Autodesk Fusion 360 part; units mm, degrees
note: some values were not read from the file. Chosen so that the rebuilt part matches the saved one: that a step has no effect; which bodies a step acts on.
(part 2 of 3)
  spline S56 degree 5 poles (56.3388, 91.0993) (56.4452, 91.2557) (56.6813, 91.5544) (57.0997, 91.9524) (57.7606, 92.3569) (58.6747, 92.6057) (59.5849, 92.5729) (60.4007, 92.2578) (61.0421, 91.6864) (61.4504, 90.9158) (61.5889, 90.0247) (61.4439, 89.103) (61.0258, 88.2423) (60.3712, 87.5263) (59.5452, 87.0208) (58.6311, 86.772) (57.7208, 86.8047) (56.905, 87.1199) (56.2637, 87.6913) (55.8554, 88.4618) (55.7168, 89.353) (55.8328, 90.0903) (56.0427, 90.6159) (56.2324, 90.9429) (56.3388, 91.0993) knots 0 0 0 0 0 0 0.05 0.1 0.15 0.2 0.25 0.3 0.35 0.4 0.45 0.5 0.55 0.6 0.65 0.7 0.75 0.8 0.85 0.9 0.95 1 1 1 1 1 1
  spline S57 degree 5 poles (56.8751, 97.0852) (56.9558, 96.9232) (57.0765, 96.5874) (57.1351, 96.0509) (56.9827, 95.2754) (56.5, 94.2116) (55.843, 93.064) (55.1256, 91.8622) (54.4274, 90.6693) (53.766, 89.5941) (53.1219, 88.7638) (52.4603, 88.2976) (51.7518, 88.283) (50.9983, 88.7439) (50.2411, 89.6329) (49.5446, 90.8558) (48.9852, 92.2891) (48.6393, 93.7983) (48.5705, 95.257) (48.8189, 96.5627) (49.3981, 97.6352) (50.2913, 98.4191) (51.4468, 98.8843) (52.7731, 99.028) (54.135, 98.8762) (55.3803, 98.4726) (56.1682, 97.9896) (56.5924, 97.5594) (56.7944, 97.2472) (56.8751, 97.0852) knots 0 0 0 0 0 0 0.04 0.08 0.12 0.16 0.2 0.24 0.28 0.32 0.36 0.4 0.44 0.48 0.52 0.56 0.6 0.64 0.68 0.72 0.76 0.8 0.84 0.88 0.92 0.96 1 1 1 1 1 1
  spline S58 degree 5 poles (71.8814, 95.613) (71.9027, 95.4116) (71.8949, 95.0024) (71.7344, 94.3767) (71.2451, 93.5503) (70.2783, 92.62) (69.0821, 91.8793) (67.7798, 91.4005) (66.4658, 91.2268) (65.1864, 91.362) (63.9606, 91.7809) (62.7952, 92.4363) (61.7022, 93.2674) (60.7152, 94.2071) (59.9065, 95.1895) (59.3667, 96.1526) (59.1837, 97.0411) (59.424, 97.8085) (60.1077, 98.4213) (61.2044, 98.8582) (62.6448, 99.107) (64.3273, 99.1623) (66.1266, 99.0235) (67.9002, 98.6914) (69.4995, 98.1694) (70.7863, 97.4683) (71.4751, 96.7812) (71.7673, 96.2113) (71.8601, 95.8145) (71.8814, 95.613) knots 0 0 0 0 0 0 0.04 0.08 0.12 0.16 0.2 0.24 0.28 0.32 0.36 0.4 0.44 0.48 0.52 0.56 0.6 0.64 0.68 0.72 0.76 0.8 0.84 0.88 0.92 0.96 1 1 1 1 1 1
  spline S59 degree 5 poles (93.1796, 92.4377) (92.9012, 92.2188) (92.3428, 91.7857) (91.5103, 91.1539) (90.4378, 90.3537) (89.1797, 89.4222) (87.9931, 88.5509) (86.8537, 87.7371) (85.7383, 86.994) (84.6458, 86.3666) (83.5926, 85.9228) (82.5959, 85.7326) (81.6625, 85.8525) (80.7707, 86.3039) (79.8819, 87.0726) (78.9677, 88.1162) (78.0294, 89.3696) (77.1277, 90.7501) (76.3717, 92.1664) (75.8904, 93.5293) (75.8092, 94.7623) (76.2256, 95.8109) (77.1816, 96.656) (78.6644, 97.3069) (80.6168, 97.79) (82.9427, 98.1396) (85.515, 98.3871) (88.1823, 98.5517) (90.7746, 98.6284) (93.1172, 98.5921) (95.0483, 98.409) (96.4351, 98.0455) (97.1913, 97.4789) (97.2921, 96.7056) (96.798, 95.7541) (95.8395, 94.6799) (94.8313, 93.7751) (94.0132, 93.0995) (93.458, 92.6567) (93.1796, 92.4377) knots 0 0 0 0 0 0 0.028571 0.057143 0.085714 0.114286 0.142857 0.171429 0.2 0.228571 0.257143 0.285714 0.314286 0.342857 0.371429 0.4 0.428571 0.457143 0.485714 0.514286 0.542857 0.571429 0.6 0.628571 0.657143 0.685714 0.714286 0.742857 0.771429 0.8 0.828571 0.857143 0.885714 0.914286 0.942857 0.971429 1 1 1 1 1 1
  line L0 (0, 0) -> (100, 0)
  line L1 (100, 0) -> (100, 100)
  line L2 (100, 100) -> (0, 100)
  line L3 (0, 100) -> (0, 0)
  point P0 (79.6579, 4.5542)
  point P1 (83.6873, 0.8119)
  point P2 (76.3709, 0.506)
  point P3 (52.7695, 4.9862)
  point P4 (57.3318, 2.811)
  point P5 (50.8771, 0.554)
  point P6 (96.4606, 14.0148)
  point P7 (98.7941, 14.2851)
  point P8 (98.8112, 7.9358)
  point P9 (92.875, 1.5897)
  point P10 (86.8955, 1.8956)
  point P11 (46.6878, 15.1123)
  point P12 (48.5368, 10.226)
  point P13 (44.8148, 3.7468)
  point P14 (39.7202, 1.5716)
  point P15 (53.9319, 10.5579)
  point P16 (52.8052, 6.5669)
  point P17 (50.0726, 10.7891)
  point P18 (80.2047, 15.9155)
  point P19 (87.817, 16.1625)
  point P20 (88.2258, 8.7488)
  point P21 (80.5937, 6.4154)
  point P22 (67.9071, 12.0123)
  point P23 (72.899, 13.9305)
  point P24 (73.8805, 11.2313)
  point P25 (70.5305, 5.4026)
  point P26 (65.0899, 1.6603)
  point P27 (60.2064, 12.5056)
  point P28 (61.4147, 5.5204)
  point P29 (60.8831, 1.6099)
  point P30 (58.7258, 3.8669)
  point P31 (55.2901, 10.0331)
  point P32 (64.2148, 19.7302)
  point P33 (68.5192, 18.2733)
  point P34 (71.0087, 16.4698)
  point P35 (67.2346, 13.716)
  point P36 (61.5672, 14.2597)
  point P37 (39.3527, 17.9605)
  point P38 (43.7129, 16.5883)
  point P39 (40.5628, 9.3364)
  point P40 (33.3674, 2.2747)
  point P41 (31.3901, 20.6466)
  point P42 (30.1837, 10.7278)
  point P43 (23.6179, 2.2941)
  point P44 (24.7173, 24.277)
  point P45 (28.0018, 24.0715)
  point P46 (23.6955, 13.0275)
  point P47 (15.6156, 3.1087)
  point P48 (19.1559, 23.32)
  point P49 (15.0058, 12.9492)
  point P50 (6.1601, 2.8249)
  point P51 (2.1097, 10.5786)
  point P52 (50.3349, 28.7902)
  point P53 (54.7428, 27.0564)
  point P54 (58.5479, 22.4518)
  point P55 (58.378, 19.3657)
  point P56 (54.9409, 17.4108)
  point P57 (51.2592, 16.9047)
  point P58 (48.2836, 17.8001)
  point P59 (46.6034, 18.5729)
  point P60 (77.4266, 28.2267)
  point P61 (80.5194, 27.0023)
  point P62 (82.2807, 22.8761)
  point P63 (79.1441, 17.9256)
  point P64 (74.5854, 16.6476)
  point P65 (73.3675, 17.4831)
  point P66 (71.9781, 29.9866)
  point P67 (73.0873, 23.6564)
  point P68 (69.5529, 19.8978)
  point P69 (15.057, 28.1496)
  point P70 (9.8735, 23.0445)
  point P71 (1.673, 21.0503)
  point P72 (91.0208, 30.4127)
  point P73 (95.3534, 23.8248)
  point P74 (95.7627, 17.1433)
  point P75 (89.3915, 18.5135)
  point P76 (84.9158, 23.217)
  point P77 (33.9696, 30.4461)
  point P78 (41.5842, 31.0743)
  point P79 (44.4066, 24.3171)
  point P80 (39.0181, 20.9457)
  point P81 (33.1247, 23.6126)
  point P82 (30.8652, 26.2228)
  point P83 (67.2233, 32.9776)
  point P84 (68.1538, 32.1594)
  point P85 (67.3369, 26.8095)
  point P86 (64.1417, 21.9362)
  point P87 (61.1337, 23.7625)
  point P88 (57.8109, 34.4437)
  point P89 (63.6671, 35.1504)
  point P90 (62.0694, 30.3434)
  point P91 (55.9996, 29.2565)
  point P92 (98.029, 32.816)
  point P93 (99.5699, 25.3331)
  point P94 (99.5529, 17.9925)
  point P95 (96.81, 24.4037)
  point P96 (16.4842, 40.0903)
  point P97 (17.8044, 42.8105)
  point P98 (19.0706, 42.1969)
  point P99 (23.606, 35.4655)
  point P100 (27.0735, 29.1141)
  point P101 (24.3862, 28.0614)
  point P102 (21.0871, 27.3883)
  point P103 (17.4249, 30.1227)
  point P104 (12.2185, 34.2787)
  point P105 (6.5411, 27.4672)
  point P106 (1.3576, 28.0394)
  point P107 (83.2708, 40.527)
  point P108 (86.6058, 36.7601)
  point P109 (85.565, 30.6337)
  point P110 (81.7651, 29.5421)
  point P111 (77.9962, 41.0906)
  point P112 (79.1698, 35.5905)
  point P113 (76.9524, 30.8901)
  point P114 (72.829, 32.0389)
  point P115 (70.1115, 33.6302)
  point P116 (7.7831, 51.8118)
  point P117 (14.5473, 46.1719)
  point P118 (13.9992, 42.5886)
  point P119 (7.2333, 38.0106)
  point P120 (1.5559, 46.472)
  point P121 (93.088, 42.9022)
  point P122 (94.9293, 37.8383)
  point P123 (94.0768, 34.227)
  point P124 (91.268, 33.3354)
  point P125 (88.2424, 37.4838)
  point P126 (36.6083, 39.904)
  point P127 (32.9758, 32.7946)
  point P128 (25.8067, 36.1809)
  point P129 (45.0765, 42.7464)
  point P130 (50.2538, 36.7891)
  point P131 (50.7512, 33.3436)
  point P132 (48.9583, 32.0429)
  point P133 (43.4327, 33.3262)
  point P134 (39.4507, 39.8074)
  point P135 (99.5711, 37.3522)
  point P136 (98.0302, 35.0244)
  point P137 (96.14, 37.703)
  point P138 (59.3387, 46.6587)
  point P139 (60.8929, 46.1985)
  point P140 (61.3985, 42.1766)
  point P141 (57.6584, 36.4209)
  point P142 (52.7347, 37.7138)
  point P143 (74.3353, 44.1904)
  point P144 (71.7761, 39.0436)
  point P145 (67.896, 35.5105)
  point P146 (65.6687, 36.7939)
  point P147 (63.5526, 41.8429)
  point P148 (96.04, 49.1785)
  point P149 (99.1607, 45.7878)
  point P150 (97.2704, 41.6705)
  point P151 (93.8882, 44.4065)
  point P152 (44.4535, 58.6502)
  point P153 (50.6119, 53.9651)
  point P154 (52.7715, 45.7846)
  point P155 (45.4083, 45.526)
  point P156 (79.0137, 56.0424)
  point P157 (82.0596, 58.6914)
  point P158 (86.8617, 53.6865)
  point P159 (89.9799, 48.3562)
  point P160 (87.3322, 45.7144)
  point P161 (83.0298, 43.5257)
  point P162 (79.475, 43.9658)
  point P163 (77.0992, 46.0034)
  point P164 (40.3762, 58.1751)
  point P165 (39.3724, 53.1339)
  point P166 (37.5699, 47.4134)
  point P167 (29.8388, 45.7456)
  point P168 (21.6709, 45.3675)
  point P169 (69.9242, 53.2274)
  point P170 (73.9562, 50.2914)
  point P171 (68.183, 47.579)
  point P172 (62.891, 47.7375)
  point P173 (25.9752, 54.1385)
  point P174 (36.1891, 59.6447)
  point P175 (28.5971, 52.2783)
  point P176 (18.5959, 46.1828)
  point P177 (17.8238, 47.0459)
  point P178 (51.7742, 62.944)
  point P179 (58.7457, 63.9787)
  point P180 (62.7216, 59.0715)
  point P181 (61.8264, 52.1149)
  point P182 (59.0452, 49.7589)
  point P183 (52.4674, 55.2104)
  point P184 (76.4459, 63.7521)
  point P185 (76.9263, 58.2048)
  point P186 (70.7568, 55.3301)
  point P187 (65.8459, 59.6129)
  point P188 (30.2252, 66.8582)
  point P189 (32.7416, 64.9211)
  point P190 (26.95, 56.7534)
  point P191 (25.1065, 65.5592)
  point P192 (22.1685, 57.8836)
  point P193 (16.3207, 49.4431)
  point P194 (9.6797, 53.9745)
  point P195 (97.2127, 66.1551)
  point P196 (98.872, 59.495)
  point P197 (95.7513, 51.889)
  point P198 (89.2508, 55.6261)
  point P199 (78.7543, 79.2824)
  point P200 (81.557, 81.7992)
  point P201 (88.0419, 75.3523)
  point P202 (88.237, 65.7773)
  point P203 (81.9734, 63.1837)
  point P204 (78.4471, 66.0821)
  point P205 (16.0982, 74.0254)
  point P206 (11.0462, 63.9161)
  point P207 (1.4654, 60.7724)
  point P208 (1.4636, 64.0146)
  point P209 (60.0445, 76.0097)
  point P210 (68.0434, 77.5129)
  point P211 (73.3977, 72.7761)
  point P212 (68.4387, 67.3518)
  point P213 (60.3971, 66.8153)
  point P214 (25.6397, 89.5124)
  point P215 (29.4587, 76.9092)
  point P216 (29.4909, 70.2325)
  point P217 (26.6373, 69.7404)
  point P218 (19.6178, 76.2868)
  point P219 (44.314, 71.0287)
  point P220 (44.5931, 62.6999)
  point P221 (42.9899, 61.8846)
  point P222 (41.6871, 61.6373)
  point P223 (39.3087, 62.9052)
  point P224 (34.9761, 66.0859)
  point P225 (32.4275, 74.6996)
  point P226 (52.3135, 78.1832)
  point P227 (54.4898, 71.1149)
  point P228 (50.5582, 66.1591)
  point P229 (46.4172, 72.2548)
  point P230 (94.8024, 80.3857)
  point P231 (98.768, 72.2616)
  point P232 (97.1087, 69.6161)
  point P233 (90.4132, 76.2607)
  point P234 (99.3391, 85.828)
  point P235 (95.3735, 82.3698)
  point P236 (52.493, 86.1688)
  point P237 (56.1856, 85.8873)
  point P238 (59.5862, 82.883)
  point P239 (58.146, 78.2422)
  point P240 (53.2824, 80.0373)
  point P241 (68.7729, 89.4265)
  point P242 (75.3354, 87.0977)
  point P243 (76.1801, 81.8417)
  point P244 (68.9433, 80.107)
  point P245 (62.3846, 83.2446)
  point P246 (15.8973, 91.7004)
  point P247 (7.2818, 78.7031)
  point P248 (2.228, 84.9448)
  point P249 (10.8389, 98.0538)
  point P250 (47.5058, 86.5545)
  point P251 (45.046, 84.5348)
  point P252 (37.3316, 84.77)
  point P253 (28.1564, 91.9777)
  point P254 (24.7262, 98.0892)
  point P255 (34.0446, 98.2008)
  point P256 (60.4137, 92.1585)
  point P257 (60.9669, 88.2783)
  point P258 (56.892, 87.2191)
  point P259 (55.1789, 91.9477)
  point P260 (52.0396, 88.3491)
  point P261 (48.755, 93.4866)
  point P262 (51.419, 98.7862)
  point P263 (67.9939, 91.5348)
  point P264 (61.7267, 93.2966)
  point P265 (59.3479, 97.3748)
  point P266 (65.1388, 99.0758)
  point P267 (86.4841, 87.5)
  point P268 (82.3055, 85.8154)
  point P269 (78.6581, 88.5545)
  point P270 (75.983, 94.9616)
  point P271 (86.3259, 98.4244)
  point P272 (97.1452, 97.1602)
move_body "Move1" bodies 2 to x (1, 0, 0) y (0, 1, 0) z (0, 0, 1) at (30, 0, 0)
extrude "Extrude12" cut sketch "Voronoi - Sketch2" along normal blind 100 contours S9 | S10 | S11 | S12 | S16 | S18 | S22 | S23 | S26 | S28 | S29 | S34 | S36 | S38 | S41 | S42 | S45 | S47 | S48 | S54 | S55 bodies 2
sketch "Voronoi - Sketch3" plane through (0, 0, 0) normal (0, 0, 1) x (1, 0, 0)
  spline S0 degree 5 poles (17.018, 3.2698) (17.8759, 3.2327) (19.5931, 3.1438) (22.1324, 2.9685) (25.2811, 2.6617) (28.4421, 2.1957) (30.5103, 1.6941) (31.2641, 1.2063) (30.6122, 0.7793) (28.634, 0.453) (25.5432, 0.2578) (21.6516, 0.2133) (17.3358, 0.3263) (13.0049, 0.5879) (9.0689, 0.9714) (5.908, 1.4374) (3.8397, 1.9391) (3.0859, 2.4269) (3.7378, 2.8538) (5.716, 3.1802) (8.8068, 3.3754) (11.9201, 3.4109) (14.446, 3.3667) (16.1602, 3.307) (17.018, 3.2698) knots 0 0 0 0 0 0 0.05 0.1 0.15 0.2 0.25 0.3 0.35 0.4 0.45 0.5 0.55 0.6 0.65 0.7 0.75 0.8 0.85 0.9 0.95 1 1 1 1 1 1
  spline S1 degree 5 poles (72.5597, 3.806) (72.5934, 4.0043) (72.6951, 4.4023) (72.9489, 4.9941) (73.475, 5.7348) (74.3766, 6.4919) (75.4317, 7.0052) (76.5375, 7.2209) (77.5882, 7.1125) (78.4845, 6.6913) (79.1407, 6.0037) (79.491, 5.1203) (79.4962, 4.128) (79.1514, 3.1214) (78.4938, 2.1955) (77.5922, 1.4385) (76.5371, 0.9251) (75.4313, 0.7094) (74.3806, 0.8179) (73.4843, 1.2391) (72.8281, 1.9267) (72.5478, 2.6334) (72.493, 3.2124) (72.526, 3.6076) (72.5597, 3.806) knots 0 0 0 0 0 0 0.05 0.1 0.15 0.2 0.25 0.3 0.35 0.4 0.45 0.5 0.55 0.6 0.65 0.7 0.75 0.8 0.85 0.9 0.95 1 1 1 1 1 1
  spline S2 degree 5 poles (84.9841, 9.4583) (85.2417, 9.591) (85.773, 9.817) (86.6121, 10.031) (87.7977, 10.0538) (89.3704, 9.67) (91.0179, 8.9401) (92.7087, 7.9558) (94.3794, 6.82) (95.9099, 5.6313) (97.1436, 4.4775) (97.9224, 3.4322) (98.1159, 2.5505) (97.6531, 1.8644) (96.5566, 1.3779) (94.9239, 1.0767) (92.9034, 0.9392) (90.6733, 0.9473) (88.4208, 1.0964) (86.3194, 1.4085) (84.5195, 1.919) (83.1417, 2.6602) (82.2682, 3.6431) (81.9355, 4.8435) (82.122, 6.1788) (82.7534, 7.5117) (83.534, 8.4519) (84.2276, 9.0208) (84.7265, 9.3256) (84.9841, 9.4583) knots 0 0 0 0 0 0 0.04 0.08 0.12 0.16 0.2 0.24 0.28 0.32 0.36 0.4 0.44 0.48 0.52 0.56 0.6 0.64 0.68 0.72 0.76 0.8 0.84 0.88 0.92 0.96 1 1 1 1 1 1
  spline S3 degree 5 poles (3.4341, 11.1117) (3.6227, 11.2638) (4.0513, 11.5485) (4.8404, 11.9144) (6.1468, 12.2844) (8.0932, 12.6168) (10.2402, 12.9058) (12.4865, 13.2242) (14.7565, 13.596) (17.0129, 13.9632) (19.24, 14.2194) (21.4267, 14.2405) (23.5492, 13.9177) (25.556, 13.1869) (27.347, 12.0663) (28.7682, 10.6723) (29.6519, 9.1712) (29.8501, 7.7412) (29.2677, 6.5339) (27.9038, 5.6283) (25.8396, 5.0394) (23.2145, 4.7403) (20.2064, 4.6793) (17.0113, 4.7989) (13.8229, 5.0528) (10.8118, 5.4269) (8.1221, 5.9283) (5.8717, 6.5707) (4.1503, 7.3615) (3.0188, 8.2864) (2.5076, 9.2982) (2.593, 10.0964) (2.9197, 10.6362) (3.2455, 10.9597) (3.4341, 11.1117) knots 0 0 0 0 0 0 0.033333 0.066667 0.1 0.133333 0.166667 0.2 0.233333 0.266667 0.3 0.333333 0.366667 0.4 0.433333 0.466667 0.5 0.533333 0.566667 0.6 0.633333 0.666667 0.7 0.733333 0.766667 0.8 0.833333 0.866667 0.9 0.933333 0.966667 1 1 1 1 1 1
  spline S4 degree 5 poles (58.3825, 7.7649) (58.3025, 8.0979) (58.1596, 8.7676) (57.9974, 9.7704) (57.8928, 11.051) (57.9754, 12.423) (58.2988, 13.4519) (58.8841, 14.0645) (59.7367, 14.2533) (60.8405, 14.0911) (62.1601, 13.6923) (63.6425, 13.1808) (65.2192, 12.6587) (66.8064, 12.1663) (68.311, 11.6809) (69.6388, 11.147) (70.7033, 10.4969) (71.4334, 9.6746) (71.7826, 8.661) (71.7356, 7.4894) (71.303, 6.2268) (70.5199, 4.961) (69.442, 3.7856) (68.1439, 2.7854) (66.7121, 2.0314) (65.2357, 1.5806) (63.7983, 1.473) (62.4696, 1.7305) (61.2961, 2.3541) (60.297, 3.3226) (59.4752, 4.5928) (58.955, 5.7982) (58.6395, 6.7693) (58.4625, 7.4319) (58.3825, 7.7649) knots 0 0 0 0 0 0 0.033333 0.066667 0.1 0.133333 0.166667 0.2 0.233333 0.266667 0.3 0.333333 0.366667 0.4 0.433333 0.466667 0.5 0.533333 0.566667 0.6 0.633333 0.666667 0.7 0.733333 0.766667 0.8 0.833333 0.866667 0.9 0.933333 0.966667 1 1 1 1 1 1
  spline S5 degree 5 poles (36.564, 13.7854) (36.7145, 13.9752) (37.0446, 14.3355) (37.6279, 14.8158) (38.5691, 15.3327) (39.9402, 15.7841) (41.4046, 16.0661) (42.8601, 16.2146) (44.2264, 16.2715) (45.4689, 16.2809) (46.5889, 16.2788) (47.6106, 16.2815) (48.5701, 16.2764) (49.5027, 16.2061) (50.4335, 15.9774) (51.3692, 15.4979) (52.2923, 14.7023) (53.1497, 13.5903) (53.8614, 12.2209) (54.3368, 10.6884) (54.4893, 9.1031) (54.2505, 7.5721) (53.5872, 6.1763) (52.5087, 4.9597) (51.0576, 3.9408) (49.3035, 3.1191) (47.3359, 2.4837) (45.2574, 2.0206) (43.1772, 1.7205) (41.204, 1.587) (39.4376, 1.6317) (37.9592, 1.8694) (36.8226, 2.3136) (36.0452, 2.9714) (35.5969, 3.8387) (35.3967, 4.8964) (35.3446, 6.1125) (35.3513, 7.4436) (35.3659, 8.8373) (35.4104, 10.2332) (35.5552, 11.5685) (35.822, 12.5416) (36.142, 13.1965) (36.4136, 13.5955) (36.564, 13.7854) knots 0 0 0 0 0 0 0.025 0.05 0.075 0.1 0.125 0.15 0.175 0.2 0.225 0.25 0.275 0.3 0.325 0.35 0.375 0.4 0.425 0.45 0.475 0.5 0.525 0.55 0.575 0.6 0.625 0.65 0.675 0.7 0.725 0.75 0.775 0.8 0.825 0.85 0.875 0.9 0.925 0.95 0.975 1 1 1 1 1 1
  spline S6 degree 5 poles (74.5422, 18.1253) (74.6384, 18.3623) (74.8439, 18.8297) (75.1897, 19.5085) (75.721, 20.3642) (76.4882, 21.3545) (77.3417, 22.2742) (78.2583, 23.1294) (79.2059, 23.9145) (80.14, 24.6034) (81.0007, 25.1405) (81.7292, 25.4593) (82.286, 25.5031) (82.6664, 25.2427) (82.9237, 24.7009) (83.1438, 23.9374) (83.411, 23.0254) (83.7715, 22.0283) (84.21, 20.9833) (84.6733, 19.9107) (85.0856, 18.8196) (85.3681, 17.7149) (85.4548, 16.6032) (85.314, 15.5007) (84.9458, 14.4318) (84.3721, 13.4247) (83.6288, 12.508) (82.7584, 11.7072) (81.8004, 11.0405) (80.7869, 10.5171) (79.7459, 10.1415) (78.7033, 9.9162) (77.6852, 9.8452) (76.7201, 9.9367) (75.841, 10.2066) (75.0814, 10.6713) (74.4717, 11.3399) (74.0349, 12.2084) (73.7824, 13.2506) (73.7141, 14.4205) (73.8221, 15.6628) (74.0385, 16.6689) (74.2668, 17.4076) (74.4461, 17.8883) (74.5422, 18.1253) knots 0 0 0 0 0 0 0.025 0.05 0.075 0.1 0.125 0.15 0.175 0.2 0.225 0.25 0.275 0.3 0.325 0.35 0.375 0.4 0.425 0.45 0.475 0.5 0.525 0.55 0.575 0.6 0.625 0.65 0.675 0.7 0.725 0.75 0.775 0.8 0.825 0.85 0.875 0.9 0.925 0.95 0.975 1 1 1 1 1 1
  spline S7 degree 5 poles (60.7414, 19.3241) (60.802, 19.5667) (60.9786, 20.0469) (61.4066, 20.7403) (62.2786, 21.5665) (63.7567, 22.338) (65.4744, 22.772) (67.2645, 22.8211) (68.9554, 22.4733) (70.3875, 21.7638) (71.4241, 20.7679) (71.9612, 19.5873) (71.9383, 18.3386) (71.3503, 17.142) (70.2604, 16.1092) (68.7823, 15.3377) (67.0646, 14.9037) (65.2745, 14.8546) (63.5836, 15.2023) (62.1515, 15.9119) (61.1149, 16.9078) (60.6853, 17.8523) (60.615, 18.5913) (60.6808, 19.0815) (60.7414, 19.3241) knots 0 0 0 0 0 0 0.05 0.1 0.15 0.2 0.25 0.3 0.35 0.4 0.45 0.5 0.55 0.6 0.65 0.7 0.75 0.8 0.85 0.9 0.95 1 1 1 1 1 1
  spline S8 degree 5 poles (92.8632, 20.9454) (93.1944, 20.8939) (93.8613, 20.7346) (94.8595, 20.3297) (96.122, 19.4813) (97.4362, 18.0178) (98.3567, 16.2984) (98.7876, 14.4901) (98.6777, 12.7661) (98.0381, 11.2894) (96.9402, 10.2014) (95.497, 9.6112) (93.8507, 9.5844) (92.1587, 10.1308) (90.5805, 11.1913) (89.2664, 12.6547) (88.3458, 14.3742) (87.9149, 16.1824) (88.0248, 17.9065) (88.6644, 19.3831) (89.7624, 20.4711) (90.9169, 20.9433) (91.8742, 21.0439) (92.532, 20.997) (92.8632, 20.9454) knots 0 0 0 0 0 0 0.05 0.1 0.15 0.2 0.25 0.3 0.35 0.4 0.45 0.5 0.55 0.6 0.65 0.7 0.75 0.8 0.85 0.9 0.95 1 1 1 1 1 1
  spline S9 degree 5 poles (10.9889, 20.653) (11.1252, 21.0131) (11.4462, 21.7388) (12.0668, 22.8271) (13.1345, 24.2083) (14.7348, 25.6557) (16.4417, 26.6835) (18.0876, 27.1857) (19.5121, 27.1031) (20.5787, 26.4389) (21.1878, 25.267) (21.2798, 23.71) (20.8405, 21.9239) (19.9064, 20.0809) (18.5717, 18.3544) (16.9714, 16.907) (15.2646, 15.8792) (13.6187, 15.377) (12.1941, 15.4596) (11.1276, 16.1238) (10.5185, 17.2957) (10.4448, 18.5412) (10.6287, 19.5786) (10.8527, 20.293) (10.9889, 20.653) knots 0 0 0 0 0 0 0.05 0.1 0.15 0.2 0.25 0.3 0.35 0.4 0.45 0.5 0.55 0.6 0.65 0.7 0.75 0.8 0.85 0.9 0.95 1 1 1 1 1 1
  spline S10 degree 5 poles (85.1604, 28.0531) (85.2638, 28.1855) (85.5042, 28.4325) (85.9654, 28.7455) (86.7772, 29.0378) (88.089, 29.1968) (89.6454, 29.1705) (91.3697, 28.9889) (93.1593, 28.6831) (94.8801, 28.275) (96.38, 27.7774) (97.5114, 27.2005) (98.1525, 26.5559) (98.2265, 25.8617) (97.7284, 25.1481) (96.7308, 24.4586) (95.3538, 23.8433) (93.744, 23.3533) (92.0505, 23.0347) (90.4014, 22.9231) (88.8837, 23.0378) (87.5551, 23.3818) (86.452, 23.9403) (85.5977, 24.6796) (85.0103, 25.5461) (84.7124, 26.4629) (84.725, 27.1657) (84.8838, 27.6382) (85.057, 27.9207) (85.1604, 28.0531) knots 0 0 0 0 0 0 0.04 0.08 0.12 0.16 0.2 0.24 0.28 0.32 0.36 0.4 0.44 0.48 0.52 0.56 0.6 0.64 0.68 0.72 0.76 0.8 0.84 0.88 0.92 0.96 1 1 1 1 1 1
  spline S11 degree 5 poles (38.1151, 22.7911) (38.0638, 23.1142) (38.0024, 23.7754) (38.0359, 24.7965) (38.3318, 26.1516) (39.0774, 27.671) (40.1234, 28.8647) (41.3699, 29.6101) (42.7004, 29.8269) (43.9882, 29.4975) (45.1075, 28.6628) (45.9453, 27.4088) (46.4136, 25.8564) (46.4623, 24.1519) (46.0925, 22.458) (45.3469, 20.9386) (44.3009, 19.7449) (43.0543, 18.9995) (41.7239, 18.7827) (40.4361, 19.1121) (39.3168, 19.9468) (38.6465, 20.95) (38.3101, 21.8367) (38.1664, 22.468) (38.1151, 22.7911) knots 0 0 0 0 0 0 0.05 0.1 0.15 0.2 0.25 0.3 0.35 0.4 0.45 0.5 0.55 0.6 0.65 0.7 0.75 0.8 0.85 0.9 0.95 1 1 1 1 1 1
  spline S12 degree 5 poles (51.3145, 24.1173) (51.3541, 24.3529) (51.4606, 24.816) (51.7016, 25.48) (52.1808, 26.2775) (53.0122, 27.0623) (54.0281, 27.5782) (55.1653, 27.7869) (56.3476, 27.6768) (57.4865, 27.2749) (58.4901, 26.6389) (59.2767, 25.841) (59.7872, 24.9543) (59.9961, 24.0393) (59.9286, 23.1269) (59.6576, 22.2162) (59.2758, 21.294) (58.8732, 20.3478) (58.5153, 19.381) (58.2139, 18.431) (57.929, 17.567) (57.5982, 16.8686) (57.1582, 16.4097) (56.5701, 16.2399) (55.8398, 16.3688) (55.0039, 16.7792) (54.1197, 17.4356) (53.2537, 18.2947) (52.471, 19.3147) (51.8321, 20.454) (51.3895, 21.6694) (51.2259, 22.6653) (51.2227, 23.4024) (51.2748, 23.8817) (51.3145, 24.1173) knots 0 0 0 0 0 0 0.033333 0.066667 0.1 0.133333 0.166667 0.2 0.233333 0.266667 0.3 0.333333 0.366667 0.4 0.433333 0.466667 0.5 0.533333 0.566667 0.6 0.633333 0.666667 0.7 0.733333 0.766667 0.8 0.833333 0.866667 0.9 0.933333 0.966667 1 1 1 1 1 1
  spline S13 degree 5 poles (46.7404, 33.2249) (46.8061, 33.2666) (46.957, 33.3095) (47.2379, 33.2553) (47.6934, 32.9696) (48.3012, 32.3342) (48.8529, 31.4935) (49.2903, 30.4851) (49.5899, 29.32) (49.7526, 28.0015) (49.7965, 26.5411) (49.7494, 24.9743) (49.6402, 23.3797) (49.4931, 21.8892) (49.3267, 20.657) (49.1529, 19.8336) (48.976, 19.5383) (48.7913, 19.8303) (48.5848, 20.685) (48.3402, 22.0165) (48.0451, 23.6958) (47.6982, 25.57) (47.3147, 27.4795) (46.9364, 29.2779) (46.6258, 30.8425) (46.4487, 32.0767) (46.458, 32.7474) (46.5629, 33.059) (46.6747, 33.1831) (46.7404, 33.2249) knots 0 0 0 0 0 0 0.04 0.08 0.12 0.16 0.2 0.24 0.28 0.32 0.36 0.4 0.44 0.48 0.52 0.56 0.6 0.64 0.68 0.72 0.76 0.8 0.84 0.88 0.92 0.96 1 1 1 1 1 1
  spline S14 degree 5 poles (26.4257, 28.757) (26.665, 28.9066) (27.1609, 29.176) (27.9507, 29.4871) (29.0636, 29.7068) (30.4653, 29.6529) (31.7893, 29.282) (32.9599, 28.618) (33.9274, 27.6938) (34.6768, 26.5489) (35.2149, 25.2293) (35.56, 23.7864) (35.7303, 22.2774) (35.7327, 20.7647) (35.5532, 19.3158) (35.1684, 17.9978) (34.5565, 16.8735) (33.7081, 15.9963) (32.6377, 15.4052) (31.3925, 15.1213) (30.0402, 15.1505) (28.6596, 15.4856) (27.3304, 16.1091) (26.1228, 16.9948) (25.0927, 18.1094) (24.2844, 19.412) (23.7308, 20.8538) (23.4552, 22.3786) (23.4717, 23.9213) (23.7858, 25.4096) (24.3914, 26.7692) (25.0933, 27.6979) (25.7255, 28.2782) (26.1865, 28.6074) (26.4257, 28.757) knots 0 0 0 0 0 0 0.033333 0.066667 0.1 0.133333 0.166667 0.2 0.233333 0.266667 0.3 0.333333 0.366667 0.4 0.433333 0.466667 0.5 0.533333 0.566667 0.6 0.633333 0.666667 0.7 0.733333 0.766667 0.8 0.833333 0.866667 0.9 0.933333 0.966667 1 1 1 1 1 1
  spline S15 degree 5 poles (6.2246, 31.1419) (6.5751, 31.3088) (7.3031, 31.6004) (8.4631, 31.9102) (10.0672, 32.0671) (11.908, 31.845) (13.3204, 31.2205) (14.0907, 30.215) (14.1252, 28.8516) (13.4613, 27.1585) (12.2213, 25.1801) (10.583, 22.9855) (8.745, 20.6782) (6.8927, 18.4078) (5.1708, 16.374) (3.6869, 14.7881) (2.5103, 13.8411) (1.6724, 13.6686) (1.1663, 14.3175) (0.9447, 15.7073) (0.9414, 17.6669) (1.0945, 19.9773) (1.3667, 22.409) (1.7734, 24.7666) (2.3846, 26.9106) (3.2833, 28.7426) (4.2847, 29.9087) (5.2004, 30.5988) (5.8741, 30.975) (6.2246, 31.1419) knots 0 0 0 0 0 0 0.04 0.08 0.12 0.16 0.2 0.24 0.28 0.32 0.36 0.4 0.44 0.48 0.52 0.56 0.6 0.64 0.68 0.72 0.76 0.8 0.84 0.88 0.92 0.96 1 1 1 1 1 1
  spline S16 degree 5 poles (63.3397, 30.3591) (63.4475, 30.6129) (63.6677, 31.1198) (64.0087, 31.8689) (64.4855, 32.8086) (65.1593, 33.7979) (65.9675, 34.5261) (66.9607, 34.9353) (68.1575, 34.9943) (69.5321, 34.7021) (71.0279, 34.0824) (72.5638, 33.1807) (74.0431, 32.0611) (75.3614, 30.8027) (76.415, 29.4973) (77.1093, 28.2399) (77.369, 27.1172) (77.1472, 26.1964) (76.4349, 25.5141) (75.2726, 25.0633) (73.7406, 24.8058) (71.9476, 24.6878) (70.0196, 24.6544) (68.0894, 24.6642) (66.2853, 24.7048) (64.7207, 24.8054) (63.4862, 25.0182) (62.6405, 25.4011) (62.2034, 26.0014) (62.1438, 26.836) (62.379, 27.8805) (62.721, 28.8406) (63.0208, 29.5968) (63.2319, 30.1053) (63.3397, 30.3591) knots 0 0 0 0 0 0 0.033333 0.066667 0.1 0.133333 0.166667 0.2 0.233333 0.266667 0.3 0.333333 0.366667 0.4 0.433333 0.466667 0.5 0.533333 0.566667 0.6 0.633333 0.666667 0.7 0.733333 0.766667 0.8 0.833333 0.866667 0.9 0.933333 0.966667 1 1 1 1 1 1
  spline S17 degree 5 poles (86.6317, 32.0032) (86.5998, 32.1461) (86.5792, 32.4458) (86.6746, 32.9333) (87.0337, 33.639) (87.7809, 34.5431) (88.7257, 35.3888) (89.7752, 36.0968) (90.8699, 36.601) (91.991, 36.8564) (93.1367, 36.8384) (94.3059, 36.5455) (95.4806, 36.0001) (96.604, 35.2523) (97.5751, 34.3772) (98.2776, 33.4603) (98.602, 32.5853) (98.4688, 31.8219) (97.857, 31.2104) (96.8093, 30.7604) (95.4128, 30.4631) (93.7865, 30.3004) (92.0673, 30.2551) (90.3961, 30.3204) (88.9056, 30.508) (87.7106, 30.8363) (87.0614, 31.2245) (86.7701, 31.588) (86.6635, 31.8602) (86.6317, 32.0032) knots 0 0 0 0 0 0 0.04 0.08 0.12 0.16 0.2 0.24 0.28 0.32 0.36 0.4 0.44 0.48 0.52 0.56 0.6 0.64 0.68 0.72 0.76 0.8 0.84 0.88 0.92 0.96 1 1 1 1 1 1
  spline S18 degree 5 poles (14.5496, 36.3223) (14.5669, 36.4572) (14.6422, 36.7264) (14.8813, 37.1314) (15.4519, 37.6874) (16.5252, 38.4388) (17.8593, 39.2653) (19.336, 40.1662) (20.8364, 41.1152) (22.2632, 42.0505) (23.5523, 42.8754) (24.6646, 43.4817) (25.5826, 43.7677) (26.3047, 43.6587) (26.8402, 43.1264) (27.2052, 42.2103) (27.418, 40.9972) (27.496, 39.5988) (27.4519, 38.131) (27.2897, 36.6916) (27.0013, 35.3392) (26.573, 34.1035) (25.9928, 32.9961) (25.2577, 32.022) (24.3793, 31.1887) (23.3941, 30.5196) (22.3614, 30.0557) (21.345, 29.8391) (20.3982, 29.8994) (19.5487, 30.2414) (18.7789, 30.8278) (18.0433, 31.5903) (17.2966, 32.4482) (16.5165, 33.3237) (15.732, 34.1597) (15.0415, 34.9337) (14.666, 35.5053) (14.5384, 35.9167) (14.5323, 36.1873) (14.5496, 36.3223) knots 0 0 0 0 0 0 0.028571 0.057143 0.085714 0.114286 0.142857 0.171429 0.2 0.228571 0.257143 0.285714 0.314286 0.342857 0.371429 0.4 0.428571 0.457143 0.485714 0.514286 0.542857 0.571429 0.6 0.628571 0.657143 0.685714 0.714286 0.742857 0.771429 0.8 0.828571 0.857143 0.885714 0.914286 0.942857 0.971429 1 1 1 1 1 1
  spline S19 degree 5 poles (48.0951, 35.231) (48.0998, 35.33) (48.139, 35.535) (48.2876, 35.8645) (48.6581, 36.3455) (49.3531, 36.9811) (50.206, 37.6015) (51.141, 38.1547) (52.1017, 38.6006) (53.0576, 38.917) (53.9954, 39.093) (54.9131, 39.1261) (55.8137, 39.017) (56.698, 38.7663) (57.5602, 38.3707) (58.387, 37.8287) (59.158, 37.1434) (59.8445, 36.3266) (60.4093, 35.4029) (60.8065, 34.4134) (60.9894, 33.41) (60.9191, 32.4499) (60.5731, 31.59) (59.9534, 30.8811) (59.0961, 30.3624) (58.0617, 30.0597) (56.922, 29.9845) (55.7493, 30.1318) (54.6045, 30.4798) (53.5235, 30.9867) (52.5155, 31.5946) (51.5767, 32.2409) (50.6997, 32.8676) (49.8853, 33.4325) (49.1515, 33.9173) (48.5486, 34.3422) (48.229, 34.6736) (48.1106, 34.9409) (48.0904, 35.132) (48.0951, 35.231) knots 0 0 0 0 0 0 0.028571 0.057143 0.085714 0.114286 0.142857 0.171429 0.2 0.228571 0.257143 0.285714 0.314286 0.342857 0.371429 0.4 0.428571 0.457143 0.485714 0.514286 0.542857 0.571429 0.6 0.628571 0.657143 0.685714 0.714286 0.742857 0.771429 0.8 0.828571 0.857143 0.885714 0.914286 0.942857 0.971429 1 1 1 1 1 1
  spline S20 degree 5 poles (37.3632, 39.5783) (37.6687, 39.5208) (38.2818, 39.3918) (39.2001, 39.1603) (40.3904, 38.7892) (41.7474, 38.2557) (42.9117, 37.6869) (43.8386, 37.1152) (44.508, 36.5721) (44.9283, 36.0856) (45.1487, 35.6825) (45.2453, 35.379) (45.2717, 35.1608) (45.2022, 34.9547) (44.9589, 34.6586) (44.4979, 34.216) (43.8239, 33.6283) (42.9699, 32.935) (41.986, 32.2022) (40.9249, 31.5078) (39.8272, 30.9278) (38.7147, 30.5265) (37.5995, 30.355) (36.4889, 30.4479) (35.3921, 30.8204) (34.3258, 31.4657) (33.3212, 32.3505) (32.4261, 33.4164) (31.6959, 34.589) (31.1873, 35.786) (30.9511, 36.9255) (31.0254, 37.9341) (31.4287, 38.7553) (32.1519, 39.3575) (33.1631, 39.7312) (34.4121, 39.8833) (35.5502, 39.8441) (36.4489, 39.7371) (37.0577, 39.6359) (37.3632, 39.5783) knots 0 0 0 0 0 0 0.028571 0.057143 0.085714 0.114286 0.142857 0.171429 0.2 0.228571 0.257143 0.285714 0.314286 0.342857 0.371429 0.4 0.428571 0.457143 0.485714 0.514286 0.542857 0.571429 0.6 0.628571 0.657143 0.685714 0.714286 0.742857 0.771429 0.8 0.828571 0.857143 0.885714 0.914286 0.942857 0.971429 1 1 1 1 1 1
  spline S21 degree 5 poles (93.421, 40.9422) (93.4382, 41.0633) (93.4929, 41.2962) (93.6338, 41.6158) (93.9243, 41.9822) (94.407, 42.3613) (94.9554, 42.6867) (95.5238, 42.9733) (96.0886, 43.2057) (96.6479, 43.3396) (97.2059, 43.3229) (97.7635, 43.1105) (98.3046, 42.6829) (98.7878, 42.0598) (99.1597, 41.288) (99.3647, 40.4334) (99.3574, 39.5718) (99.1124, 38.78) (98.6384, 38.1269) (97.9739, 37.668) (97.1769, 37.4431) (96.3177, 37.4712) (95.4699, 37.7472) (94.702, 38.2362) (94.0715, 38.876) (93.6231, 39.5922) (93.4332, 40.1664) (93.3901, 40.5696) (93.4039, 40.8211) (93.421, 40.9422) knots 0 0 0 0 0 0 0.04 0.08 0.12 0.16 0.2 0.24 0.28 0.32 0.36 0.4 0.44 0.48 0.52 0.56 0.6 0.64 0.68 0.72 0.76 0.8 0.84 0.88 0.92 0.96 1 1 1 1 1 1
  spline S22 degree 5 poles (70.897, 38.0452) (70.9299, 38.1518) (71.0391, 38.3547) (71.3314, 38.6286) (71.9613, 38.9336) (73.0691, 39.2137) (74.3954, 39.3889) (75.8317, 39.4528) (77.2774, 39.397) (78.6573, 39.2101) (79.923, 38.881) (81.045, 38.402) (82.008, 37.7719) (82.8049, 37.0005) (83.4319, 36.1104) (83.8817, 35.1434) (84.1459, 34.1537) (84.2226, 33.1967) (84.1238, 32.3169) (83.8811, 31.539) (83.5561, 30.8521) (83.2226, 30.2267) (82.9372, 29.643) (82.7156, 29.114) (82.5009, 28.716) (82.198, 28.5498) (81.7192, 28.6883) (81.018, 29.1399) (80.0812, 29.8688) (78.9268, 30.808) (77.5994, 31.8748) (76.1673, 32.985) (74.7191, 34.0682) (73.3592, 35.0795) (72.1957, 35.9925) (71.3292, 36.7955) (70.9396, 37.3487) (70.8416, 37.7151) (70.8641, 37.9386) (70.897, 38.0452) knots 0 0 0 0 0 0 0.028571 0.057143 0.085714 0.114286 0.142857 0.171429 0.2 0.228571 0.257143 0.285714 0.314286 0.342857 0.371429 0.4 0.428571 0.457143 0.485714 0.514286 0.542857 0.571429 0.6 0.628571 0.657143 0.685714 0.714286 0.742857 0.771429 0.8 0.828571 0.857143 0.885714 0.914286 0.942857 0.971429 1 1 1 1 1 1
  spline S23 degree 5 poles (70.2184, 43.6537) (70.2083, 43.7999) (70.2374, 44.0931) (70.429, 44.5282) (70.9706, 45.0705) (72.0508, 45.6194) (73.4257, 45.9838) (74.9625, 46.1245) (76.5159, 46.0257) (77.9383, 45.7003) (79.0922, 45.1835) (79.8613, 44.527) (80.1633, 43.7937) (79.9631, 43.0529) (79.2861, 42.3751) (78.2059, 41.8262) (76.831, 41.4618) (75.2942, 41.321) (73.7408, 41.4199) (72.3184, 41.7452) (71.1645, 42.262) (70.5492, 42.7873) (70.2979, 43.2157) (70.2285, 43.5074) (70.2184, 43.6537) knots 0 0 0 0 0 0 0.05 0.1 0.15 0.2 0.25 0.3 0.35 0.4 0.45 0.5 0.55 0.6 0.65 0.7 0.75 0.8 0.85 0.9 0.95 1 1 1 1 1 1
  spline S24 degree 5 poles (63.0539, 43.5604) (63.1655, 43.7902) (63.3934, 44.2472) (63.7453, 44.9189) (64.2214, 45.7631) (64.8049, 46.6734) (65.3613, 47.3856) (65.8811, 47.8583) (66.3584, 48.0682) (66.7892, 48.0158) (67.1687, 47.731) (67.4938, 47.2606) (67.7631, 46.6569) (67.9794, 45.9638) (68.1485, 45.2146) (68.2772, 44.4344) (68.3714, 43.6417) (68.4343, 42.8504) (68.4644, 42.0711) (68.4551, 41.3126) (68.3953, 40.5828) (68.2693, 39.8896) (68.0577, 39.2418) (67.7365, 38.6501) (67.2837, 38.1273) (66.6872, 37.6884) (65.9521, 37.3502) (65.1094, 37.1317) (64.2211, 37.0535) (63.3643, 37.135) (62.6193, 37.3918) (62.0559, 37.8327) (61.7202, 38.4576) (61.6221, 39.2541) (61.7454, 40.1995) (62.0547, 41.2617) (62.4139, 42.1725) (62.7238, 42.8683) (62.9423, 43.3306) (63.0539, 43.5604) knots 0 0 0 0 0 0 0.028571 0.057143 0.085714 0.114286 0.142857 0.171429 0.2 0.228571 0.257143 0.285714 0.314286 0.342857 0.371429 0.4 0.428571 0.457143 0.485714 0.514286 0.542857 0.571429 0.6 0.628571 0.657143 0.685714 0.714286 0.742857 0.771429 0.8 0.828571 0.857143 0.885714 0.914286 0.942857 0.971429 1 1 1 1 1 1
  spline S25 degree 5 poles (54.3281, 43.1129) (54.3768, 43.2814) (54.5098, 43.6213) (54.8135, 44.132) (55.409, 44.7821) (56.3942, 45.4666) (57.5214, 45.9564) (58.681, 46.2008) (59.7614, 46.1714) (60.6597, 45.8691) (61.2906, 45.3278) (61.591, 44.6039) (61.5269, 43.7699) (61.1002, 42.9058) (60.3557, 42.0932) (59.3706, 41.4087) (58.2433, 40.9189) (57.0838, 40.6745) (56.0034, 40.7039) (55.105, 41.0062) (54.4742, 41.5475) (54.2339, 42.1266) (54.2176, 42.6105) (54.2795, 42.9444) (54.3281, 43.1129) knots 0 0 0 0 0 0 0.05 0.1 0.15 0.2 0.25 0.3 0.35 0.4 0.45 0.5 0.55 0.6 0.65 0.7 0.75 0.8 0.85 0.9 0.95 1 1 1 1 1 1
  spline S26 degree 5 poles (5.6572, 47.7618) (5.8821, 47.6875) (6.3295, 47.4769) (6.9871, 46.982) (7.8222, 46.0149) (8.7842, 44.487) (9.6635, 42.8578) (10.4563, 41.3275) (11.1438, 40.04) (11.6763, 39.0352) (11.9669, 38.2259) (11.9271, 37.4839) (11.493, 36.7006) (10.6623, 35.8746) (9.4944, 35.109) (8.0881, 34.555) (6.567, 34.3715) (5.0617, 34.6804) (3.6936, 35.5177) (2.568, 36.8446) (1.7691, 38.5642) (1.3542, 40.5354) (1.3477, 42.5876) (1.7349, 44.5346) (2.4545, 46.1881) (3.4166, 47.379) (4.2987, 47.8586) (4.9797, 47.9225) (5.4322, 47.836) (5.6572, 47.7618) knots 0 0 0 0 0 0 0.04 0.08 0.12 0.16 0.2 0.24 0.28 0.32 0.36 0.4 0.44 0.48 0.52 0.56 0.6 0.64 0.68 0.72 0.76 0.8 0.84 0.88 0.92 0.96 1 1 1 1 1 1
  spline S27 degree 5 poles (28.3951, 46.4988) (28.4516, 46.5618) (28.6022, 46.683) (28.94, 46.8527) (29.5975, 47.0686) (30.6783, 47.3527) (31.9115, 47.6724) (33.1934, 48.0294) (34.446, 48.3967) (35.6381, 48.7111) (36.7667, 48.8929) (37.8431, 48.862) (38.8765, 48.5567) (39.8602, 47.9494) (40.7523, 47.0691) (41.4818, 45.9952) (41.9676, 44.8347) (42.1346, 43.7055) (41.9302, 42.718) (41.3425, 41.9545) (40.4101, 41.4576) (39.2037, 41.2389) (37.8132, 41.2848) (36.333, 41.5624) (34.8485, 42.0256) (33.4212, 42.6211) (32.0959, 43.2924) (30.9069, 43.9848) (29.8847, 44.6494) (29.0631, 45.2479) (28.4842, 45.7569) (28.2645, 46.0899) (28.2634, 46.3046) (28.3387, 46.4357) (28.3951, 46.4988) knots 0 0 0 0 0 0 0.033333 0.066667 0.1 0.133333 0.166667 0.2 0.233333 0.266667 0.3 0.333333 0.366667 0.4 0.433333 0.466667 0.5 0.533333 0.566667 0.6 0.633333 0.666667 0.7 0.733333 0.766667 0.8 0.833333 0.866667 0.9 0.933333 0.966667 1 1 1 1 1 1
  spline S28 degree 5 poles (83.1608, 48.4367) (83.2945, 48.5255) (83.5845, 48.6717) (84.0861, 48.7952) (84.8748, 48.7677) (86.0008, 48.4407) (87.1903, 47.8679) (88.3597, 47.1054) (89.4278, 46.2086) (90.3265, 45.2214) (91.0034, 44.1777) (91.4216, 43.1062) (91.5618, 42.0334) (91.4227, 40.9877) (91.0232, 40.0037) (90.4016, 39.1232) (89.6087, 38.3895) (88.7025, 37.8414) (87.7425, 37.5093) (86.7832, 37.4079) (85.8708, 37.5355) (85.0413, 37.8803) (84.3185, 38.4242) (83.7126, 39.1479) (83.2181, 40.0348) (82.8219, 41.0664) (82.5104, 42.2173) (82.2773, 43.4509) (82.1298, 44.715) (82.0981, 45.9357) (82.2242, 47.0285) (82.4844, 47.7347) (82.7823, 48.1393) (83.027, 48.348) (83.1608, 48.4367) knots 0 0 0 0 0 0 0.033333 0.066667 0.1 0.133333 0.166667 0.2 0.233333 0.266667 0.3 0.333333 0.366667 0.4 0.433333 0.466667 0.5 0.533333 0.566667 0.6 0.633333 0.666667 0.7 0.733333 0.766667 0.8 0.833333 0.866667 0.9 0.933333 0.966667 1 1 1 1 1 1
  spline S29 degree 5 poles (47.0013, 47.5363) (47.1568, 47.6385) (47.4771, 47.8309) (47.9804, 48.0821) (48.6722, 48.3376) (49.4996, 48.5082) (50.2235, 48.5148) (50.7975, 48.3491) (51.2111, 48.0154) (51.5023, 47.5355) (51.7305, 46.9426) (51.9518, 46.2743) (52.1919, 45.567) (52.4249, 44.8496) (52.5965, 44.1434) (52.6438, 43.4607) (52.5138, 42.8044) (52.1875, 42.1658) (51.6831, 41.5285) (51.0411, 40.8775) (50.3145, 40.2069) (49.558, 39.5276) (48.8158, 38.877) (48.1136, 38.3226) (47.4645, 37.9432) (46.8735, 37.8124) (46.3418, 37.9825) (45.8722, 38.4644) (45.4716, 39.222) (45.1498, 40.1905) (44.919, 41.2878) (44.7934, 42.4293) (44.7886, 43.5401) (44.9211, 44.5714) (45.2048, 45.4966) (45.6472, 46.3049) (46.1249, 46.8566) (46.5443, 47.2174) (46.8459, 47.4341) (47.0013, 47.5363) knots 0 0 0 0 0 0 0.028571 0.057143 0.085714 0.114286 0.142857 0.171429 0.2 0.228571 0.257143 0.285714 0.314286 0.342857 0.371429 0.4 0.428571 0.457143 0.485714 0.514286 0.542857 0.571429 0.6 0.628571 0.657143 0.685714 0.714286 0.742857 0.771429 0.8 0.828571 0.857143 0.885714 0.914286 0.942857 0.971429 1 1 1 1 1 1
  spline S30 degree 5 poles (14.4362, 47.0165) (14.5944, 47.226) (14.9277, 47.6278) (15.4744, 48.1718) (16.2815, 48.7589) (17.3825, 49.2417) (18.5384, 49.4783) (19.7129, 49.4934) (20.8705, 49.3268) (21.9768, 49.0277) (22.9978, 48.649) (23.8993, 48.2395) (24.645, 47.8357) (25.1964, 47.455) (25.5097, 47.0847) (25.5415, 46.6863) (25.2621, 46.2183) (24.6704, 45.6566) (23.7918, 44.9984) (22.6718, 44.2583) (21.3714, 43.4681) (19.9616, 42.6748) (18.5183, 41.9395) (17.1175, 41.3359) (15.8314, 40.9396) (14.7251, 40.8171) (13.8523, 41.0149) (13.2521, 41.5495) (12.9441, 42.3936) (12.9268, 43.4728) (13.1832, 44.6856) (13.5841, 45.6716) (13.9786, 46.3707) (14.278, 46.807) (14.4362, 47.0165) knots 0 0 0 0 0 0 0.033333 0.066667 0.1 0.133333 0.166667 0.2 0.233333 0.266667 0.3 0.333333 0.366667 0.4 0.433333 0.466667 0.5 0.533333 0.566667 0.6 0.633333 0.666667 0.7 0.733333 0.766667 0.8 0.833333 0.866667 0.9 0.933333 0.966667 1 1 1 1 1 1
  spline S31 degree 5 poles (7.5784, 54.0416) (7.9079, 53.809) (8.5563, 53.3239) (9.482, 52.548) (10.5623, 51.466) (11.5278, 50.168) (12.0118, 49.0547) (11.9594, 48.2394) (11.3674, 47.8053) (10.2976, 47.7892) (8.8624, 48.1866) (7.207, 48.9568) (5.4936, 50.0282) (3.8865, 51.3016) (2.5362, 52.6541) (1.5707, 53.9521) (1.0867, 55.0654) (1.139, 55.8806) (1.7311, 56.3148) (2.8009, 56.3308) (4.2361, 55.9335) (5.5604, 55.3173) (6.5798, 54.7197) (7.249, 54.2742) (7.5784, 54.0416) knots 0 0 0 0 0 0 0.05 0.1 0.15 0.2 0.25 0.3 0.35 0.4 0.45 0.5 0.55 0.6 0.65 0.7 0.75 0.8 0.85 0.9 0.95 1 1 1 1 1 1
  spline S32 degree 5 poles (96.4819, 54.1995) (96.4818, 54.7357) (96.4972, 55.8104) (96.5673, 57.4035) (96.7511, 59.387) (97.1063, 61.3928) (97.5514, 62.7234) (98.0433, 63.2369) (98.5355, 62.8717) (98.9812, 61.6731) (99.3374, 59.7709) (99.5683, 57.3575) (99.6489, 54.6663) (99.5696, 51.9525) (99.34, 49.4731) (98.9847, 47.4674) (98.5396, 46.1367) (98.0477, 45.6233) (97.5555, 45.9884) (97.1098, 47.1871) (96.7536, 49.0892) (96.5689, 51.02) (96.498, 52.593) (96.482, 53.6632) (96.4819, 54.1995) knots 0 0 0 0 0 0 0.05 0.1 0.15 0.2 0.25 0.3 0.35 0.4 0.45 0.5 0.55 0.6 0.65 0.7 0.75 0.8 0.85 0.9 0.95 1 1 1 1 1 1
  spline S33 degree 5 poles (85.8552, 55.516) (85.8543, 55.7176) (85.8846, 56.1156) (86.0265, 56.7002) (86.4022, 57.4684) (87.1423, 58.4376) (88.0928, 59.4226) (89.1797, 60.398) (90.3196, 61.2876) (91.4278, 61.9755) (92.4289, 62.3367) (93.2662, 62.2611) (93.9127, 61.6823) (94.3785, 60.5982) (94.6955, 59.058) (94.9059, 57.1527) (95.0494, 55.0056) (95.1514, 52.7625) (95.2079, 50.5828) (95.1886, 48.6272) (95.0508, 47.0418) (94.7495, 45.9442) (94.2492, 45.4079) (93.5349, 45.4473) (92.6244, 46.0011) (91.5613, 46.9568) (90.4081, 48.1763) (89.2391, 49.5206) (88.1339, 50.8763) (87.1707, 52.1755) (86.4204, 53.3843) (86.0373, 54.2748) (85.89, 54.906) (85.8561, 55.3144) (85.8552, 55.516) knots 0 0 0 0 0 0 0.033333 0.066667 0.1 0.133333 0.166667 0.2 0.233333 0.266667 0.3 0.333333 0.366667 0.4 0.433333 0.466667 0.5 0.533333 0.566667 0.6 0.633333 0.666667 0.7 0.733333 0.766667 0.8 0.833333 0.866667 0.9 0.933333 0.966667 1 1 1 1 1 1
  spline S34 degree 5 poles (53.2339, 50.7356) (53.2707, 50.8914) (53.3583, 51.2004) (53.5307, 51.6527) (53.8392, 52.2228) (54.3549, 52.8684) (55.001, 53.4415) (55.7753, 53.9376) (56.6679, 54.3467) (57.6583, 54.6488) (58.7183, 54.8206) (59.8136, 54.8406) (60.9069, 54.6945) (61.9593, 54.3803) (62.933, 53.9151) (63.7929, 53.3357) (64.5076, 52.6887) (65.0498, 52.0231) (65.3977, 51.3818) (65.5357, 50.794) (65.4555, 50.2673) (65.1562, 49.7961) (64.6447, 49.3678) (63.9362, 48.9705) (63.0538, 48.5957) (62.0273, 48.2397) (60.8929, 47.9045) (59.6921, 47.6001) (58.4713, 47.3454) (57.2812, 47.1701) (56.1724, 47.108) (55.1918, 47.1907) (54.3782, 47.4413) (53.7586, 47.8678) (53.3434, 48.4559) (53.1244, 49.166) (53.0917, 49.7902) (53.1376, 50.2656) (53.1971, 50.5798) (53.2339, 50.7356) knots 0 0 0 0 0 0 0.028571 0.057143 0.085714 0.114286 0.142857 0.171429 0.2 0.228571 0.257143 0.285714 0.314286 0.342857 0.371429 0.4 0.428571 0.457143 0.485714 0.514286 0.542857 0.571429 0.6 0.628571 0.657143 0.685714 0.714286 0.742857 0.771429 0.8 0.828571 0.857143 0.885714 0.914286 0.942857 0.971429 1 1 1 1 1 1
  spline S35 degree 5 poles (39.7135, 51.1726) (39.7318, 51.2513) (39.7833, 51.4044) (39.9043, 51.6195) (40.1524, 51.8727) (40.6083, 52.1249) (41.207, 52.3047) (41.9338, 52.4031) (42.7529, 52.4074) (43.6131, 52.3045) (44.4538, 52.0846) (45.2112, 51.7453) (45.8247, 51.2952) (46.2426, 50.7579) (46.4291, 50.177) (46.3654, 49.6082) (46.0515, 49.1085) (45.5069, 48.7278) (44.7731, 48.4971) (43.9115, 48.4254) (42.9935, 48.5057) (42.0933, 48.7187) (41.2797, 49.0374) (40.6081, 49.4307) (40.1118, 49.8679) (39.7977, 50.3213) (39.6857, 50.6776) (39.6733, 50.932) (39.6951, 51.0939) (39.7135, 51.1726) knots 0 0 0 0 0 0 0.04 0.08 0.12 0.16 0.2 0.24 0.28 0.32 0.36 0.4 0.44 0.48 0.52 0.56 0.6 0.64 0.68 0.72 0.76 0.8 0.84 0.88 0.92 0.96 1 1 1 1 1 1
  spline S36 degree 5 poles (69.5474, 55.1072) (69.6377, 55.2411) (69.8268, 55.504) (70.1367, 55.8828) (70.604, 56.352) (71.2821, 56.8659) (72.0563, 57.2955) (72.9259, 57.6316) (73.8863, 57.8696) (74.9278, 58.0092) (76.0342, 58.0521) (77.1822, 58.0005) (78.3399, 57.8543) (79.4657, 57.61) (80.5065, 57.2578) (81.4043, 56.7857) (82.1043, 56.1848) (82.5623, 55.4543) (82.7522, 54.6062) (82.6754, 53.6715) (82.3552, 52.6952) (81.8279, 51.728) (81.1352, 50.82) (80.3168, 50.0134) (79.4005, 49.3341) (78.4027, 48.7917) (77.3343, 48.3852) (76.2057, 48.1067) (75.0315, 47.9459) (73.8351, 47.8942) (72.6552, 47.9496) (71.5414, 48.1156) (70.5454, 48.3969) (69.7131, 48.7962) (69.0773, 49.311) (68.6483, 49.9292) (68.4109, 50.628) (68.3363, 51.3798) (68.3909, 52.1559) (68.5475, 52.9324) (68.7918, 53.6928) (69.0526, 54.2786) (69.2852, 54.7008) (69.4571, 54.9734) (69.5474, 55.1072) knots 0 0 0 0 0 0 0.025 0.05 0.075 0.1 0.125 0.15 0.175 0.2 0.225 0.25 0.275 0.3 0.325 0.35 0.375 0.4 0.425 0.45 0.475 0.5 0.525 0.55 0.575 0.6 0.625 0.65 0.675 0.7 0.725 0.75 0.775 0.8 0.825 0.85 0.875 0.9 0.925 0.95 0.975 1 1 1 1 1 1
  spline S37 degree 5 poles (45.7155, 54.0686) (45.7749, 54.129) (45.9176, 54.236) (46.2009, 54.3528) (46.6989, 54.4172) (47.4532, 54.3473) (48.2593, 54.1395) (49.0379, 53.8137) (49.7224, 53.3952) (50.2727, 52.9113) (50.6807, 52.3898) (50.9568, 51.8589) (51.1203, 51.3462) (51.1889, 50.8783) (51.1677, 50.4807) (51.0417, 50.1765) (50.7906, 49.9853) (50.3991, 49.9214) (49.8709, 49.9918) (49.2283, 50.1962) (48.5072, 50.527) (47.7545, 50.9685) (47.0246, 51.4969) (46.3761, 52.08) (45.8686, 52.6764) (45.5559, 53.241) (45.4935, 53.6318) (45.5612, 53.8736) (45.6561, 54.0082) (45.7155, 54.0686) knots 0 0 0 0 0 0 0.04 0.08 0.12 0.16 0.2 0.24 0.28 0.32 0.36 0.4 0.44 0.48 0.52 0.56 0.6 0.64 0.68 0.72 0.76 0.8 0.84 0.88 0.92 0.96 1 1 1 1 1 1
  spline S38 degree 5 poles (11.8726, 66.474) (12.3659, 66.5463) (13.3509, 66.6758) (14.8075, 66.8218) (16.6533, 66.904) (18.7004, 66.7661) (20.4219, 66.3345) (21.7812, 65.5698) (22.7671, 64.4586) (23.3902, 63.0301) (23.6765, 61.3531) (23.6591, 59.5237) (23.372, 57.6573) (22.8412, 55.8784) (22.0796, 54.3111) (21.0918, 53.0677) (19.8784, 52.2368) (18.4405, 51.8728) (16.7838, 51.9813) (14.9249, 52.5249) (12.8981, 53.4365) (10.7625, 54.6295) (8.608, 56.0091) (6.565, 57.4832) (4.8033, 58.9714) (3.4992, 60.4055) (2.8083, 61.7322) (2.8379, 62.9144) (3.6153, 63.934) (5.0667, 64.7928) (7.0512, 65.5019) (8.9195, 65.9591) (10.391, 66.2418) (11.3793, 66.4017) (11.8726, 66.474) knots 0 0 0 0 0 0 0.033333 0.066667 0.1 0.133333 0.166667 0.2 0.233333 0.266667 0.3 0.333333 0.366667 0.4 0.433333 0.466667 0.5 0.533333 0.566667 0.6 0.633333 0.666667 0.7 0.733333 0.766667 0.8 0.833333 0.866667 0.9 0.933333 0.966667 1 1 1 1 1 1
  spline S39 degree 5 poles (40.1507, 61.267) (40.1518, 61.5969) (40.155, 62.2562) (40.1618, 63.2358) (40.1797, 64.4946) (40.2533, 65.934) (40.4251, 67.1958) (40.7368, 68.2433) (41.2103, 69.0425) (41.8313, 69.5575) (42.5368, 69.7473) (43.2459, 69.5808) (43.8837, 69.0486) (44.4133, 68.1806) (44.8314, 67.0386) (45.1529, 65.7022) (45.3988, 64.2575) (45.584, 62.7848) (45.7022, 61.3448) (45.7205, 59.9726) (45.597, 58.6891) (45.2928, 57.5097) (44.7872, 56.4542) (44.0899, 55.5544) (43.2605, 54.8671) (42.397, 54.466) (41.6045, 54.4195) (40.9711, 54.774) (40.5355, 55.5303) (40.2837, 56.6423) (40.1724, 58.0334) (40.1504, 59.2937) (40.1484, 60.277) (40.1496, 60.9371) (40.1507, 61.267) knots 0 0 0 0 0 0 0.033333 0.066667 0.1 0.133333 0.166667 0.2 0.233333 0.266667 0.3 0.333333 0.366667 0.4 0.433333 0.466667 0.5 0.533333 0.566667 0.6 0.633333 0.666667 0.7 0.733333 0.766667 0.8 0.833333 0.866667 0.9 0.933333 0.966667 1 1 1 1 1 1
  spline S40 degree 5 poles (32.5035, 65.6323) (32.7871, 65.8268) (33.3644, 66.2008) (34.2511, 66.713) (35.4271, 67.2726) (36.7451, 67.6786) (37.7814, 67.705) (38.448, 67.288) (38.7378, 66.4135) (38.7349, 65.1277) (38.5679, 63.5173) (38.3745, 61.6962) (38.2648, 59.7897) (38.2779, 57.9197) (38.3624, 56.1915) (38.4171, 54.6883) (38.3195, 53.4634) (37.9592, 52.5337) (37.2691, 51.872) (36.2578, 51.3999) (34.9892, 51.019) (33.5614, 50.6452) (32.0866, 50.2369) (30.6691, 49.837) (29.3936, 49.5664) (28.3252, 49.5692) (27.5062, 49.9735) (26.9538, 50.8417) (26.6583, 52.1344) (26.594, 53.7472) (26.7288, 55.5396) (27.0337, 57.3672) (27.4926, 59.1115) (28.1124, 60.7133) (28.9121, 62.1576) (29.9089, 63.4544) (30.866, 64.3883) (31.6626, 65.0342) (32.2198, 65.4379) (32.5035, 65.6323) knots 0 0 0 0 0 0 0.028571 0.057143 0.085714 0.114286 0.142857 0.171429 0.2 0.228571 0.257143 0.285714 0.314286 0.342857 0.371429 0.4 0.428571 0.457143 0.485714 0.514286 0.542857 0.571429 0.6 0.628571 0.657143 0.685714 0.714286 0.742857 0.771429 0.8 0.828571 0.857143 0.885714 0.914286 0.942857 0.971429 1 1 1 1 1 1
  spline S41 degree 5 poles (46.8318, 69.5483) (46.9253, 69.6359) (47.1385, 69.7747) (47.5351, 69.8744) (48.1989, 69.8027) (49.1692, 69.4292) (50.1839, 68.8371) (51.1634, 68.0779) (52.0646, 67.1751) (52.8663, 66.1374) (53.5607, 64.9673) (54.1418, 63.6724) (54.597, 62.2741) (54.8933, 60.82) (54.9855, 59.3798) (54.8311, 58.0338) (54.4036, 56.8645) (53.7053, 55.947) (52.7836, 55.3392) (51.7367, 55.0743) (50.6809, 55.1656) (49.7253, 55.6081) (48.9442, 56.3811) (48.3495, 57.4507) (47.9106, 58.7707) (47.574, 60.2835) (47.2831, 61.9209) (46.9969, 63.605) (46.7109, 65.2486) (46.4722, 66.7569) (46.3535, 68.0389) (46.4158, 68.8219) (46.5773, 69.2491) (46.7383, 69.4607) (46.8318, 69.5483) knots 0 0 0 0 0 0 0.033333 0.066667 0.1 0.133333 0.166667 0.2 0.233333 0.266667 0.3 0.333333 0.366667 0.4 0.433333 0.466667 0.5 0.533333 0.566667 0.6 0.633333 0.666667 0.7 0.733333 0.766667 0.8 0.833333 0.866667 0.9 0.933333 0.966667 1 1 1 1 1 1
  spline S42 degree 5 poles (58.214, 68.9054) (58.4099, 68.9819) (58.823, 69.0819) (59.5021, 69.0681) (60.5037, 68.7203) (61.8494, 67.7916) (63.2141, 66.4675) (64.5178, 64.8735) (65.6781, 63.1465) (66.6123, 61.4176) (67.2434, 59.8029) (67.5093, 58.4012) (67.3718, 57.2883) (66.8246, 56.5138) (65.9059, 56.0938) (64.6976, 56.0131) (63.3058, 56.2393) (61.8462, 56.7351) (60.4263, 57.4707) (59.1319, 58.4338) (58.0305, 59.6155) (57.1723, 60.9993) (56.5922, 62.5477) (56.3111, 64.1918) (56.3375, 65.814) (56.6674, 67.2624) (57.1611, 68.1583) (57.6477, 68.6226) (58.0181, 68.8288) (58.214, 68.9054) knots 0 0 0 0 0 0 0.04 0.08 0.12 0.16 0.2 0.24 0.28 0.32 0.36 0.4 0.44 0.48 0.52 0.56 0.6 0.64 0.68 0.72 0.76 0.8 0.84 0.88 0.92 0.96 1 1 1 1 1 1
  spline S43 degree 5 poles (67.626, 74.6103) (67.8302, 74.7015) (68.2584, 74.8126) (68.9502, 74.7602) (69.9278, 74.2527) (71.1186, 72.961) (72.1571, 71.1415) (72.9372, 68.9675) (73.3834, 66.6442) (73.4596, 64.3945) (73.163, 62.4379) (72.5221, 60.9708) (71.5943, 60.1459) (70.464, 60.0508) (69.2421, 60.6851) (68.0513, 61.9768) (67.0128, 63.7963) (66.2327, 65.9704) (65.7865, 68.2937) (65.7103, 70.5434) (66.0069, 72.5) (66.5196, 73.6737) (67.0333, 74.2649) (67.4218, 74.519) (67.626, 74.6103) knots 0 0 0 0 0 0 0.05 0.1 0.15 0.2 0.25 0.3 0.35 0.4 0.45 0.5 0.55 0.6 0.65 0.7 0.75 0.8 0.85 0.9 0.95 1 1 1 1 1 1